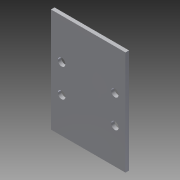
# Autodesk Inventor part: Aluminum Plate (0.125)
Saved by Autodesk Inventor 2014 (Build 180170000, 170)
## iProperties
Created: 2014-01-18
Part Number: Aluminum Plate (0.125)
Material: Aluminum 6061
Document SubType Name: Modeling
Designer: Andrew Toennies
Mass: 20.5908 g
Surface Area: 57.0457 cm^2
Volume: 7.59807 cm^3
Density: 2.71 g/cm^3
Appearance: Aluminum - Flat
Author: Andrew Toennies
Autodesk Inventor part; units mm, degrees
ref_plane "YZ Plane" through (0, 0, 0) normal (1, 0, 0) x (0, 1, 0)
ref_plane "XZ Plane" through (0, 0, 0) normal (0, 1, 0) x (-1, 0, 0)
ref_plane "XY Plane" through (0, 0, 0) normal (0, 0, 1) x (1, 0, 0)
sketch "Sketch1" plane through (0, 0, 0) normal (0, 0, 1) x (1, 0, 0)
  line L0 (66.802, 0) -> (66.802, 38.1)
  line L1 (0, 38.1) -> (0, 0)
  line L2 (9.525, 31.75) -> (57.277, 31.75) construction
  line L3 (57.277, 31.75) -> (57.277, 6.35) construction
  line L4 (57.277, 6.35) -> (9.525, 6.35) construction
  line L5 (9.525, 6.35) -> (9.525, 31.75) construction
  circle A0 centre (9.525, 31.75) radius 3.3782
  circle A1 centre (9.525, 6.35) radius 3.3782
  circle A2 centre (57.277, 31.75) radius 3.3782
  circle A3 centre (57.277, 6.35) radius 3.3782
  line L6 (0, 0) -> (0, -25.4)
  line L7 (0, -25.4) -> (66.802, -25.4)
  line L8 (66.802, -25.4) -> (66.802, 0)
  line L9 (0, 38.1) -> (0, 76.2)
  line L10 (0, 76.2) -> (66.802, 76.2)
  line L11 (66.802, 76.2) -> (66.802, 38.1)
  point P0 (0, 0)
  dimension "d0" = 38.1
  dimension "d1" = 66.802
  dimension "d2" = 25.4
  dimension "d3" = 47.752
  dimension "d4" = 9.525
  dimension "d6" = 6.7564
  dimension "d7" = 6.7564
  dimension "d8" = 6.7564
  dimension "d9" = 6.7564
  dimension "d14" = 6.35
  dimension "d15" = 9.525
  dimension "d17" = 25.4
  dimension "d18" = 101.6
  constraints: 24 end point, 6 parallel, 4 centre point, 4 coincident, 3 perpendicular, 1 collinear, 1 horizontal, 1 point on line
  measures "d0" distance of L1.start point (0, 0)
  measures "d1" distance of L0.end L1.start
  measures "d2" distance of L4.end L2.start
  measures "d3" distance of L2.start L2.end
  measures "d4" distance between parallel lines of L0 L3
  measures "d6" diameter of A0
  measures "d7" diameter of A1
  measures "d8" diameter of A2
  measures "d9" diameter of A3
  measures "d14" distance from line of L2 L1.start
  measures "d15" distance between parallel lines of L1 L5
  measures "d17" distance from line of point (0, 0) L7
  measures "d18" distance between parallel lines of L7 L10
extrude "Extrusion1" add sketch "Sketch1" along normal blind 3.175
sketch "Sketch3" plane through (0, 0, 3.175) normal (0, 0, 1) x (1, 0, 0)
  circle A0 centre (44.3929, -15.875) radius 2.0701
  circle A1 centre (44.3929, 60.325) radius 2.0701
  line L0 (46.463, -25.4) -> (46.463, -23.114)
  point P0 (0, 0)
  dimension "d25" = 4.1402
  dimension "d26" = 4.1402
  dimension "d27" = 9.525
  dimension "d28" = 76.2
  constraints: 2 centre point, 2 end point, 2 tangent, 1 vertical, 2 other
  measures "d25" diameter of A0
  measures "d26" diameter of A1
  measures "d27" vertical distance of L0.start A0.centre
  measures "d28" distance of A1.centre A0.centre
extrude "Extrusion3" cut sketch "Sketch3" against normal blind 25.4
equation "\"d4\" = -0.5 * d3 + 0.5 * d1"
body "Solid1"
